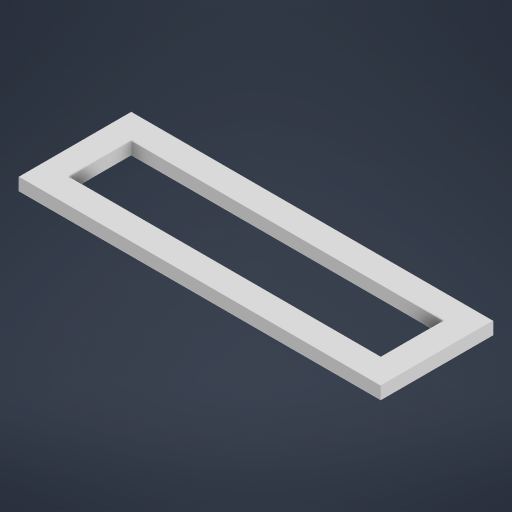
# Autodesk Inventor part: Langbektang houder
Saved by Autodesk Inventor 2023.2 (Build 272271000, 271)
## iProperties
Created: 2020-09-09
Part Number: Langbektang houder
Material: Generic
Document SubType Name: Modeling
Designer: nathan.bollaert
Density: 1 g/cm^3
Appearance: Default
Author: nathan.bollaert
Autodesk Inventor part; units mm, degrees
ref_plane "YZ Plane" through (0, 0, 0) normal (1, 0, 0) x (0, 1, 0)
ref_plane "XZ Plane" through (0, 0, 0) normal (0, 1, 0) x (-1, 0, 0)
ref_plane "XY Plane" through (0, 0, 0) normal (0, 0, 1) x (1, 0, 0)
sketch "Sketch1" plane through (0, 0, 0) normal (0, 1, 0) x (-1, 0, 0)
  line L0 (-50, 10) -> (50, 10)
  line L1 (50, 10) -> (50, -10)
  line L2 (50, -10) -> (-50, -10)
  line L3 (-50, -10) -> (-50, 10)
  line L4 (-50, 10) -> (50, -10) construction
  line L5 (50, 10) -> (-50, -10) construction
  line L6 (-50, 10) -> (50, 10) construction
  line L7 (-58, -18) -> (58, -18)
  line L8 (58, -18) -> (58, 18)
  line L9 (58, 18) -> (-58, 18)
  line L10 (-58, 18) -> (-58, -18)
  line L11 (-58, -18) -> (58, 18) construction
  line L12 (58, -18) -> (-58, 18) construction
  point P0 (0, 0)
  dimension "d230" = 100
  dimension "d232" = 20
  dimension "d234" = 8
  dimension "d235" = 8
  constraints: 26 end point, 4 midpoint, 4 parallel, 3 horizontal, 2 perpendicular, 1 collinear
  measures "d230" distance of L0.start L0.end
  measures "d232" distance of L0.end L1.end
  measures "d234" distance between parallel lines of L8 L1
  measures "d235" distance between parallel lines of L0 L9
extrude "Extrusion1" add sketch "Sketch1" along normal blind 4
body "Solid5"
